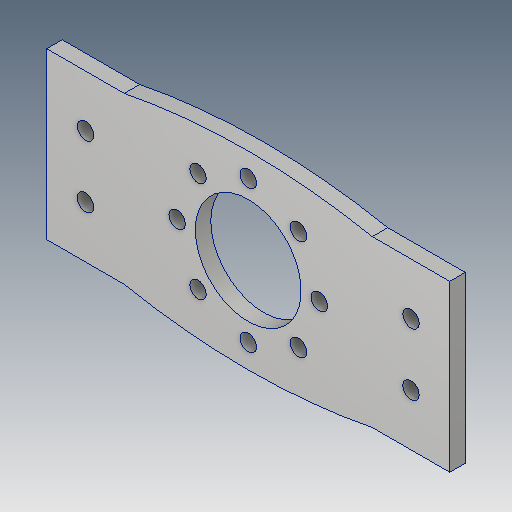
# Autodesk Inventor part: サーボ支え板B_アルミ(A2017)_t3
Saved by Autodesk Inventor 2019.4 (Build 234330000, 330)
## iProperties
Created: 2019-06-16
Part Number: サーボ支え板B_アルミ(A2017)_t3
Material: アルミニウム 6061
Document SubType Name: Modeling
Designer: 長谷川翔一
Mass: 19.957 g
Surface Area: 57.083 cm^2
Volume: 7.39149 cm^3
Density: 2.7 g/cm^3
Appearance: アルミニウム - フラット
Author: 長谷川翔一
Autodesk Inventor part; units mm, degrees
ref_plane "YZ Plane" through (0, 0, 0) normal (1, 0, 0) x (0, 1, 0)
ref_plane "XZ Plane" through (0, 0, 0) normal (0, 1, 0) x (-1, 0, 0)
ref_plane "XY Plane" through (0, 0, 0) normal (0, 0, 1) x (1, 0, 0)
sketch "スケッチ1" plane through (0, 0, 0) normal (0, 0, 1) x (1, 0, 0)
  line L0 (-39, -16) -> (-39, 16)
  line L1 (39, 16) -> (39, -16)
  line L2 (39, -16) -> (-39, 16) construction
  line L3 (-39, -16) -> (39, 16) construction
  line L4 (0, 0) -> (0, 16) construction
  line L5 (0, 0) -> (-39, 0) construction
  line L6 (-39, 16) -> (-24, 16)
  line L7 (-24, 16) -> (-24, -16) construction
  line L8 (-31.5, 16) -> (-31.5, -16) construction
  line L9 (-24, 0) -> (-39, 0) construction
  circle A0 centre (-31.5, 6) radius 1.6
  circle A1 centre (-31.5, -6) radius 1.6
  line L10 (24, 16) -> (24, -16) construction
  line L11 (31.5, 16) -> (31.5, -16) construction
  line L12 (24, 0) -> (39, 0) construction
  circle A2 centre (31.5, 6) radius 1.6
  circle A3 centre (31.5, -6) radius 1.6
  line L13 (-39, 16) -> (-24, 16)
  line L14 (24, 16) -> (39, 16)
  line L15 (39, -16) -> (24, -16)
  line L16 (-24, -16) -> (-39, -16)
  circle A4 centre (0, 0) radius 13.75
  circle A5 centre (0, 13.75) radius 1.6
  circle A6 centre (0, -13.75) radius 1.6
  arc A7 (24, 16) -> (-24, 16) centre (0, -105.3782) ccw
  arc A8 (-24, -16) -> (24, -16) centre (0, 105.3782) ccw
  dimension "d5" = 78
  dimension "d6" = 32
  dimension "d7" = 15
  dimension "d8" = 3.2
  dimension "d9" = 6
  dimension "d44" = 27.5
  dimension "d45" = 3.2
  dimension "d46" = 3.2
  dimension "d47" = 3
  dimension "d48" = 3
  constraints: 34 end point, 9 centre point, 9 symmetric about line, 7 perpendicular, 6 midpoint, 6 point on circle, 5 parallel, 3 point on line, 2 horizontal, 1 coincident, 3 other
  measures "d5" distance of L0.end L1.start
  measures "d6" distance of L0.start L0.end
  measures "d7" distance of L0.end L6.end
  measures "d8" diameter of A0
  measures "d9" distance from line of A0.centre L5
  measures "d44" diameter of A4
  measures "d45" diameter of A5
  measures "d46" diameter of A6
extrude "押し出し2" add sketch "スケッチ1" along normal blind 3 contours L0 L6 A7 L14 L1 L15 A8 L16 | A4 A6 A5 | A5 A4 | A4 A5 | A6 A4 | A4 A6
sketch "スケッチ4" plane through (0, 0, 0) normal (0, 0, -1) x (-1, 0, 0)
  circle A0 centre (-31.5, 6) radius 1.6 projected
  circle A1 centre (-31.5, -6) radius 1.6 projected
  circle A2 centre (31.5, -6) radius 1.6 projected
  circle A3 centre (31.5, 6) radius 1.6 projected
  line L0 (24, 16) -> (39, 16) projected
  line L1 (-39, 16) -> (-24, 16) projected
  line L2 (-39, -16) -> (-39, 16) projected
  line L3 (-24, -16) -> (-39, -16) projected
  line L4 (39, -16) -> (24, -16) projected
  line L5 (39, 16) -> (39, -16) projected
  line L6 (-39, 0) -> (39, 0) construction
  line L7 (0, 36) -> (0, -36) construction
  circle A4 centre (0, 0) radius 10.25
  circle A5 centre (0, 0) radius 13.75 construction
  circle A6 centre (0, 13.75) radius 1.6
  circle A7 centre (0, 0) radius 13.75 construction
  circle A8 centre (-9.7227, 9.7227) radius 1.6
  circle A9 centre (0, 0) radius 13.75 construction
  circle A10 centre (-13.75, 0) radius 1.6
  circle A11 centre (0, 0) radius 13.75 construction
  circle A12 centre (-9.7227, -9.7227) radius 1.6
  circle A13 centre (0, 0) radius 13.75 construction
  circle A14 centre (0, -13.75) radius 1.6
  circle A15 centre (0, 0) radius 13.75 construction
  circle A16 centre (9.7227, -9.7227) radius 1.6
  circle A17 centre (0, 0) radius 13.75 construction
  circle A18 centre (13.75, 0) radius 1.6
  circle A19 centre (0, 0) radius 13.75 construction
  circle A20 centre (9.7227, 9.7227) radius 1.6
  arc A21 (24, 16) -> (-24, 16) centre (0, -105.3782) ccw projected
  arc A22 (-24, -16) -> (24, -16) centre (0, 105.3782) ccw projected
  dimension "d17" = 27.5
  dimension "d16" = 20.5
  dimension "d18" = 3.2
  dimension "d21" = 360
  constraints: 9 centre point, 4 end point, 2 coincident, 2 horizontal alignment, 2 midpoint, 2 vertical alignment, 1 point on line, 53 other
  measures "d16" diameter of A4
  measures "d18" diameter of A6
extrude "押し出し4" cut sketch "スケッチ4" against normal through all contours A4 | A6 | A8 | A10 | A12 | A14 | A16 | A18 | A20
